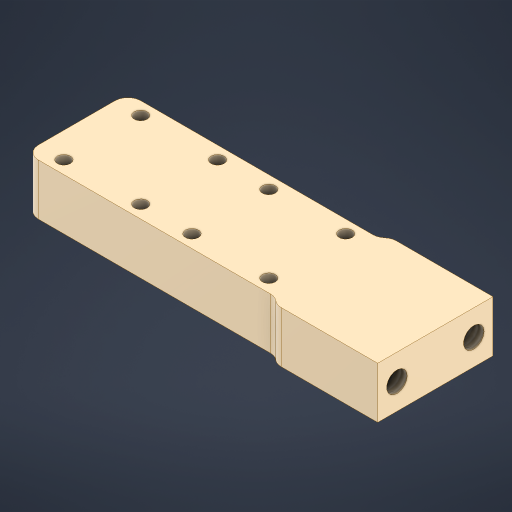
# Autodesk Inventor part: DVBS_009_RemoteLookingBracket
Saved by Autodesk Inventor 2024.2 (Build 282272000, 272)
## iProperties
Created: 2024-08-10
Part Number: DVBS_009_RemoteLookingBracket
Material: Polyethylene, High Density
Document SubType Name: Modeling
Designer: Bryan
Density: 0.952 g/cm^3
Appearance: Smooth - Off-White
Author: Bryan
Autodesk Inventor part; units mm, degrees
ref_plane "YZ Plane" through (0, 0, 0) normal (1, 0, 0) x (0, 1, 0)
ref_plane "XZ Plane" through (0, 0, 0) normal (0, 1, 0) x (-1, 0, 0)
ref_plane "XY Plane" through (0, 0, 0) normal (0, 0, 1) x (1, 0, 0)
sketch "Sketch1" plane through (0, 0, 0) normal (0, 1, 0) x (-1, 0, 0)
  line L0 (0, 0) -> (63.5, 0)
  line L1 (63.5, 0) -> (63.5, -25.4)
  line L2 (63.5, -25.4) -> (0, -25.4)
  line L3 (0, -25.4) -> (0, 0) construction
  line L4 (0, 1.5875) -> (-25.4, 1.5875)
  line L5 (-25.4, 1.5875) -> (-25.4, -26.9875)
  line L6 (-25.4, -26.9875) -> (0, -26.9875)
  line L7 (0, -26.9875) -> (0, 1.5875)
  circle A0 centre (6.35, -3.175) radius 1.6256
  circle A1 centre (25.4, -3.175) radius 1.6256
  circle A2 centre (6.35, -22.225) radius 1.6256
  circle A3 centre (25.4, -22.225) radius 1.6256
  circle A4 centre (57.15, -3.175) radius 1.6256
  circle A5 centre (57.15, -22.225) radius 1.6256
  circle A6 centre (38.1, -3.175) radius 1.6256
  circle A7 centre (38.1, -22.225) radius 1.6256
  point P0 (0, -12.7)
  point P1 (0, -12.7)
  point P2 (-12.7, 1.5875)
  point P3 (-12.7, -26.9875)
  point P4 (0, -25.4)
  dimension "d0" = 25.4
  dimension "d11" = 63.5
  dimension "d12" = 25.4
  dimension "d20" = 3.2512
  dimension "d23" = 19.05
  dimension "d26" = 19.05
  dimension "d29" = 3.2512
  dimension "d32" = 19.05
  dimension "d35" = 19.05
  dimension "d38" = 12.7
  dimension "d39" = 6.35
  dimension "d40" = 3.175
  dimension "d41" = 28.575
  constraints: 16 end point, 8 centre point, 4 horizontal, 4 midpoint, 4 parallel, 2 perpendicular, 2 vertical, 1 coincident, 1 collinear, 1 horizontal alignment, 12 other
  measures "d0" distance of L5.end L6.end
  measures "d11" distance of L1.end L2.end
  measures "d12" distance of L0.end L1.end
  measures "d20" diameter of A0
  measures "d23" distance of A0.centre A1.centre
  measures "d26" distance of A0.centre A2.centre
  measures "d29" diameter of A4
  measures "d32" distance of A4.centre A5.centre
  measures "d35" distance of A4.centre A6.centre
  measures "d38" distance of A1.centre A6.centre
  measures "d39" distance from line of L3 A0.centre
  measures "d40" distance from line of L0 A0.centre
  measures "d41" distance of L4.end L5.end
extrude "Extrusion1" add sketch "Sketch1" along normal blind 12.7
fillet "Fillet1" radius 3.175 6 edges at (-63.5, 6.35, -25.4) (-63.5, 6.35, 0) (0, 6.35, -25.4) (0, 6.35, -26.9875) (0, 6.35, 0) (0, 6.35, 1.5875)
sketch "Sketch2" plane through (25.4, 0, 1.5875) normal (1, 0, 0) x (0, 0, -1)
  line L0 (0, 12.7) -> (28.575, 12.7)
  line L1 (28.575, 12.7) -> (28.575, 0)
  line L2 (28.575, 0) -> (0, 0)
  line L3 (0, 0) -> (0, 12.7)
  line L4 (0, 12.7) -> (28.575, 0) construction
  line L5 (28.575, 12.7) -> (0, 0) construction
  line L6 (0, 12.7) -> (28.575, 12.7) projected
  line L7 (0, 0) -> (0, 12.7) projected
  circle A0 centre (23.8125, 6.35) radius 2.5527
  circle A1 centre (4.7625, 6.35) radius 2.5527
  point P0 (1.5875, 0)
  point P1 (14.2875, 6.35)
  dimension "d45" = 5.1054
  dimension "d46" = 9.525
  dimension "d47" = 9.525
  constraints: 12 end point, 2 centre point, 2 collinear, 2 horizontal alignment, 2 midpoint, 2 parallel, 1 coincident, 1 equal radius, 1 horizontal, 1 perpendicular
  measures "d45" diameter of A0
  measures "d46" distance of point (14.288, 6.35) A0.centre
  measures "d47" distance of A1.centre point (14.288, 6.35)
extrude "Extrusion2" cut sketch "Sketch2" against normal blind 25.4 contours A0 | A1
thread "Thread1" size "1/4-20 UNC" class "2B" standard "ANSI Unified Screw Threads" full length
thread "Thread2" size "1/4-20 UNC" class "2B" standard "ANSI Unified Screw Threads" full length
body "Solid1"
